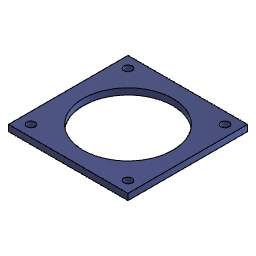
bearing_top_cap (Autodesk Fusion 360 design; units mm, degrees)
Autodesk Fusion 360 part; units mm, degrees
sketch "Sketch1" plane through (0, 0, 0) normal (0, 1, 0) x (1, 0, 0)
  line L0 (-24, 24) -> (24, 24)
  line L1 (24, 24) -> (24, -24)
  line L2 (24, -24) -> (-24, -24)
  line L3 (-24, -24) -> (-24, 24)
  circle A0 centre (0, 0) radius 18
  circle A1 centre (19.5, -19.5) radius 1.65
  circle A2 centre (19.5, 19.5) radius 1.65
  circle A3 centre (-19.5, 19.5) radius 1.65
  circle A4 centre (-19.5, -19.5) radius 1.65
  dimension "d1" = 24
  dimension "d2" = 48
  dimension "d3" = 24
  dimension "d4" = 48
  dimension "d7" = 36
  dimension "d8" = 3.3
  dimension "d9" = 19.5
  dimension "d10" = 19.5
  dimension "d13" = 360
  constraint horizontal L0
  constraint vertical L1
  constraint horizontal L2
  constraint vertical L3
  constraint coincident A0.centre origin
  measures "d1" distance of A0.centre L0
  measures "d2" distance of L0.start L2.end
  measures "d3" distance of A0.centre L1
  measures "d4" distance of L1.end L2.end
  measures "d7" diameter of A0
  measures "d8" diameter of A1
  measures "d9" horizontal distance of A0.centre A1.centre
  measures "d10" vertical distance of A0.centre A1.centre
extrude "Extrude1" add sketch "Sketch1" along normal blind 2.5
equation "d1 = size / 2"
equation "d2 = size"
equation "d3 = size / 2"
equation "d4 = size"
equation "d9 = ( 39 / 2 ) * 1 mm"
equation "d10 = ( 39 / 2 ) * 1 mm"
equation "size = 48 mm"
